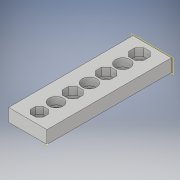
# Autodesk Inventor part: multiplebolts
Saved by Autodesk Inventor 2019 (Build 230136000, 136)
## iProperties
Created: 2018-12-20
Part Number: multiplebolts
Material: Generic
Document SubType Name: Modeling
Designer: assman
Density: 1 g/cm^3
Appearance: Default
Author: assman
## iProperties of the stored document multiplebolts_3DPrint.ipt
Created: 2018-12-20
Part Number: multiplebolts_3DPrint
Material: Generic
Document SubType Name: Modeling
Designer: assman
Density: 1 g/cm^3
Appearance: Default
Author: assman
Autodesk Inventor part; units mm, degrees
ref_plane "YZ Plane" through (0, 0, 0) normal (1, 0, 0) x (0, 1, 0)
ref_plane "XZ Plane" through (0, 0, 0) normal (0, 1, 0) x (-1, 0, 0)
ref_plane "XY Plane" through (0, 0, 0) normal (0, 0, 1) x (1, 0, 0)
sketch "Sketch1" plane through (0, 0, 0) normal (0, 1, 0) x (-1, 0, 0)
  line L0 (15, 0) -> (0, 0)
  line L1 (0, 0) -> (0, -50)
  line L2 (0, -50) -> (15, -50)
  line L3 (15, -50) -> (15, 0)
  dimension "d0" = 15
  dimension "d1" = 50
  constraints: 8 end point, 2 parallel, 1 coincident, 1 horizontal, 1 perpendicular
  measures "d0" distance of L2.end L1.end
  measures "d1" distance of L1.end L0.end
extrude "Extrusion1" add sketch "Sketch1" along normal blind 5
sketch "Sketch2" plane through (0, 5, 0) normal (0, 1, 0) x (1, 0, 0)
  line L0 (-15, 50) -> (-15, 0) construction
  line L1 (-15, 0) -> (0, 0) construction
  line L2 (0, 0) -> (0, 50) construction
  line L3 (0, 50) -> (-15, 50) construction
  line L4 (-15, 50) -> (-15, 0) construction
  line L5 (-15, 0) -> (0, 0) construction
  line L6 (-7.5, 0) -> (-7.5, 50) construction
  line L7 (0, 50) -> (-15, 50) construction
  line L8 (-15, 25) -> (0, 25) construction
  line L9 (-4.9593, 5.6025) -> (-4.9593, 3.4978)
  line L10 (-4.9593, 3.4978) -> (-6.4476, 2.0095)
  line L11 (-6.4476, 2.0095) -> (-8.5524, 2.0095)
  line L12 (-8.5524, 2.0095) -> (-10.0407, 3.4978)
  line L13 (-10.0407, 3.4978) -> (-10.0407, 5.6025)
  line L14 (-10.0407, 5.6025) -> (-8.5524, 7.0908)
  line L15 (-8.5524, 7.0908) -> (-6.4476, 7.0908)
  line L16 (-6.4476, 7.0908) -> (-4.9593, 5.6025)
  line L17 (-15, 2.0095) -> (0, 2.0095) construction
  line L18 (0, 0) -> (0, 50) construction
  line L19 (-10.4, 16.3489) -> (-10.4, 18.7514)
  line L20 (-10.4, 18.7514) -> (-8.7012, 20.4502)
  line L21 (-8.7012, 20.4502) -> (-6.2988, 20.4502)
  line L22 (-6.2988, 20.4502) -> (-4.6, 18.7514)
  line L23 (-4.6, 18.7514) -> (-4.6, 16.3489)
  line L24 (-4.6, 16.3489) -> (-6.2988, 14.6502)
  line L25 (-6.2988, 14.6502) -> (-8.7012, 14.6502)
  line L26 (-8.7012, 14.6502) -> (-10.4, 16.3489)
  line L27 (-7.5, 4.5502) -> (-7.5, 17.5502) construction
  circle A0 centre (-7.5, 11.0502) radius 2.75
  line L28 (-7.5, 17.5502) -> (-7.5, 30.5502) construction
  circle A1 centre (-7.5, 24.0502) radius 2.825
  line L29 (-4.55, 31.7721) -> (-4.55, 29.3282)
  line L30 (-4.55, 29.3282) -> (-6.2781, 27.6002)
  line L31 (-6.2781, 27.6002) -> (-8.7219, 27.6002)
  line L32 (-8.7219, 27.6002) -> (-10.45, 29.3282)
  line L33 (-10.45, 29.3282) -> (-10.45, 31.7721)
  line L34 (-10.45, 31.7721) -> (-8.7219, 33.5002)
  line L35 (-8.7219, 33.5002) -> (-6.2781, 33.5002)
  line L36 (-6.2781, 33.5002) -> (-4.55, 31.7721)
  line L37 (-7.5, 30.5502) -> (-7.5, 43.5502) construction
  circle A2 centre (-7.5, 37.0502) radius 2.85
  line L38 (-4.5, 44.7928) -> (-4.5, 42.3075)
  line L39 (-4.5, 42.3075) -> (-6.2574, 40.5502)
  line L40 (-6.2574, 40.5502) -> (-8.7426, 40.5502)
  line L41 (-8.7426, 40.5502) -> (-10.5, 42.3075)
  line L42 (-10.5, 42.3075) -> (-10.5, 44.7928)
  line L43 (-10.5, 44.7928) -> (-8.7426, 46.5502)
  line L44 (-8.7426, 46.5502) -> (-6.2574, 46.5502)
  line L45 (-6.2574, 46.5502) -> (-4.5, 44.7928)
  line L46 (-15, 46.5502) -> (0, 46.5502) construction
  line L47 (-15, 48.5597) -> (0, 48.5597) construction
  dimension "d12" = 2.0095
  dimension "d14" = 2.5407
  dimension "d15" = 2.9
  dimension "d17" = 5.5
  dimension "d18" = 5.65
  dimension "d19" = 2.95
  dimension "d20" = 5.7
  dimension "d21" = 3
  dimension "d22" = 2.0095
  constraints: 80 end point, 6 point on line, 4 collinear, 4 midpoint, 4 parallel, 3 centre point, 3 perpendicular, 1 coincident, 20 other
  measures "d12" distance between parallel lines of L1 L17
  measures "d14" distance from line of L27.start L10
  measures "d15" distance from line of L27.end L24
  measures "d17" diameter of A0
  measures "d18" diameter of A1
  measures "d19" distance from line of L30 L37.start
  measures "d20" diameter of A2
  measures "d21" distance from line of point (-7.5, 43.55) L39
  measures "d22" distance between parallel lines of L46 L47
ref_plane "Work Plane1" through (-15, 5, -48.5597) normal (0, 0, 1) x (1, 0, 0)
split "Split1" plane through (-15, 5, -48.5597) removes the side toward (0, 0, -1)
extrude "Extrusion2" cut sketch "Sketch2" against normal blind 2.85 contours L9 L10 L11 L12 L13 L14 L15 L16
extrude "Extrusion6" cut sketch "Sketch2" against normal blind 2.85 contours A0
extrude "Extrusion3" cut sketch "Sketch2" against normal blind 3 contours L19 L20 L21 L22 L23 L24 L25 L26
extrude "Extrusion7" cut sketch "Sketch2" against normal blind 3 contours A1
extrude "Extrusion4" cut sketch "Sketch2" against normal blind 3.05 contours L29 L30 L31 L32 L33 L34 L35 L36
extrude "Extrusion5" cut sketch "Sketch2" against normal blind 3.1 contours L38 L39 L40 L41 L42 L43 L44 L45
hole "Hole2" at (-7.5, 5, -4.5502) direction (0, -1, 0) diameter 3.121 end through all thread size "M3.5x0.35" class "6H" standard "ISO Metric profile"
hole "Hole3" at (-7.5, 5, -11.0502) direction (0, -1, 0) diameter 3.121 end through all thread size "M3.5x0.35" class "6H" standard "ISO Metric profile"
hole "Hole4" at (-7.5, 5, -17.5502) direction (0, -1, 0) diameter 3.242 end through all thread size "M4x0.7" class "6H" standard "ISO Metric profile"
hole "Hole5" at (-7.5, 5, -24.0502) direction (0, -1, 0) diameter 3.242 end through all thread size "M4x0.7" class "6H" standard "ISO Metric profile"
hole "Hole6" at (-7.5, 5, -30.5502) direction (0, -1, 0) diameter 3.459 end through all thread size "M4x0.5" class "6H" standard "ISO Metric profile"
extrude "Extrusion8" cut sketch "Sketch2" against normal blind 3.1 contours A2
sketch "Sketch4" plane through (-7.5, 1.9, -37.0502) normal (0, 1, 0) x (1, 0, 0)
  circle A0 centre (0, 0) radius 2.85 construction
  line L0 (0, 0) -> (0, 2.85) construction
  line L1 (-1.5605, -0.6464) -> (-1.5605, 0.6464)
  line L2 (-1.5605, 0.6464) -> (-0.6464, 1.5605)
  line L3 (-0.6464, 1.5605) -> (0.6464, 1.5605)
  line L4 (0.6464, 1.5605) -> (1.5605, 0.6464)
  line L5 (1.5605, 0.6464) -> (1.5605, -0.6464)
  line L6 (1.5605, -0.6464) -> (0.6464, -1.5605)
  line L7 (0.6464, -1.5605) -> (-0.6464, -1.5605)
  line L8 (-0.6464, -1.5605) -> (-1.5605, -0.6464)
  point P0 (7.5, -37.0502)
  dimension "d81" = 1.5605
  constraints: 18 end point, 1 coincident, 1 parallel, 1 vertical, 1 vertical alignment, 18 other
  measures "d81" distance from line of L0.start L8
sketch "Sketch5" plane through (0, 0, 0) normal (0, -1, 0) x (1, 0, 0)
  point P0 (0, 0)
extrude "Extrusion9" cut sketch "Sketch4" against normal blind 3.1
sketch "Sketch6" plane through (0, 1.9, 0) normal (0, 1, 0) x (1, 0, 0)
  line L0 (-4.5, 44.7928) -> (-4.5, 42.3075) construction
  line L1 (-6.2574, 46.5502) -> (-4.5, 44.7928) construction
  line L2 (-8.7426, 46.5502) -> (-6.2574, 46.5502) construction
  line L3 (-10.5, 44.7928) -> (-8.7426, 46.5502) construction
  line L4 (-10.5, 42.3075) -> (-10.5, 44.7928) construction
  line L5 (-8.7426, 40.5502) -> (-10.5, 42.3075) construction
  line L6 (-6.2574, 40.5502) -> (-8.7426, 40.5502) construction
  line L7 (-4.5, 42.3075) -> (-6.2574, 40.5502) construction
  line L8 (-4.5, 42.3075) -> (-6.2574, 40.5502) construction
  line L9 (-4.5, 42.3075) -> (-10.5, 44.7928) construction
  line L10 (-10.5, 42.3075) -> (-10.5, 44.7928) construction
  line L11 (-6.2574, 46.5502) -> (-4.5, 44.7928) construction
  line L12 (-10.5, 42.3075) -> (-4.5, 44.7928) construction
  line L13 (-7.5, 43.5502) -> (-7.5, 46.5502) construction
  line L14 (-7.5, 46.5502) -> (-7.5, 40.5502) construction
  line L15 (-6.2574, 40.5502) -> (-8.7426, 40.5502) construction
  line L16 (-9.2105, 42.8416) -> (-9.2105, 44.2587)
  line L17 (-9.2105, 44.2587) -> (-8.2085, 45.2607)
  line L18 (-8.2085, 45.2607) -> (-6.7915, 45.2607)
  line L19 (-6.7915, 45.2607) -> (-5.7895, 44.2587)
  line L20 (-5.7895, 44.2587) -> (-5.7895, 42.8416)
  line L21 (-5.7895, 42.8416) -> (-6.7915, 41.8397)
  line L22 (-6.7915, 41.8397) -> (-8.2085, 41.8397)
  line L23 (-8.2085, 41.8397) -> (-9.2105, 42.8416)
  point P0 (0, 0)
  dimension "d84" = 1.7105
  constraints: 24 end point, 3 midpoint, 2 point on line, 1 coincident, 17 other
  measures "d84" distance from line of L13.start L23
extrude "Extrusion10" cut sketch "Sketch6" against normal blind 3.1
thread "Thread2" size "M3.5x0.6" class "6H" standard "ANSI Metric M Profile" full length
thread "Thread3" size "M3.5x0.6" class "6H" standard "ANSI Metric M Profile" full length
sketch "Sketch8" plane through (-7.5, 2.15, -11.0502) normal (1, 0, 0) x (0, 0, 1)
  line L0 (1.5605, 0) -> (1.5605, 2.15)
  line L1 (1.5605, 2.15) -> (1.1156, 2.15)
  line L2 (1.1156, 2.15) -> (1.1156, 0)
  line L3 (1.1156, 0) -> (1.5605, 0)
  line L4 (0, -3.85) -> (0, 3.15) projected
  constraints: 8 end point
revolve "Revolution1" add sketch "Sketch8" angle 360 about axis through (-7.5, 2.15, -11.0502) along (0, -1, 0) separate body
sketch "Sketch7" plane through (-7.5, 2.15, -9.4897) normal (-1, 0, 0) x (0, -1, 0)
  line L0 (-0.3501, -0.0305) -> (-0.3001, -0.0305) construction
  line L1 (0.0499, -0.4147) -> (-0.0001, -0.5108) construction
  line L2 (-0.6001, -0.5108) -> (-0.6501, -0.4147) construction
  line L3 (-0.2501, -0.0305) -> (-0.3001, 0.0655) construction
  line L4 (-0.3001, 0.0655) -> (-0.3501, -0.0305) construction
  line L5 (-0.6001, -0.5108) -> (-0.5501, -0.4147) construction
  line L6 (-0.2501, -0.0305) -> (-0.0501, -0.4147)
  line L7 (-0.6501, -0.4147) -> (-0.5501, -0.4147) construction
  arc A0 (-0.6501, -0.4147) -> (-0.6001, -0.445) centre (-0.6001, -0.3887) ccw construction
  line L8 (0.0499, -0.4147) -> (-0.0501, -0.4147) construction
  line L9 (-0.6001, -0.5108) -> (-0.6001, -0.4147) construction
  line L10 (-0.0001, -0.5108) -> (-0.0001, -0.4147) construction
  line L11 (-0.3001, 0.0655) -> (-0.3001, -0.0002) construction
  line L12 (-0.6001, -0.445) -> (-0.0001, -0.445)
  arc A1 (-0.6001, -0.445) -> (-0.5501, -0.4147) centre (-0.6001, -0.3887) ccw
  line L13 (-0.0501, -0.4147) -> (-0.0001, -0.5108) construction
  line L14 (-0.5501, -0.4147) -> (-0.3501, -0.0305)
  line L15 (-0.0001, -0.0002) -> (-0.0001, 0.0177)
  line L16 (-0.0001, 0.0177) -> (-0.0001, -0.0002)
  line L17 (-0.0001, -0.0002) -> (0.0334, -0.0002)
  arc A2 (-0.0501, -0.4147) -> (-0.0001, -0.445) centre (-0.0001, -0.3887) ccw
  arc A3 (-0.0001, -0.445) -> (0.0499, -0.4147) centre (-0.0001, -0.3887) ccw construction
  arc A4 (-0.3001, -0.0002) -> (-0.3501, -0.0305) centre (-0.3001, -0.0565) ccw
  arc A5 (-0.2501, -0.0305) -> (-0.3001, -0.0002) centre (-0.3001, -0.0565) ccw
  line L18 (-0.3001, -0.0002) -> (-0.3001, -0.0305) construction
  line L19 (-0.3001, -0.0305) -> (-0.2501, -0.0305) construction
  dimension "d93" = 55
  dimension "d94" = 0.096
  dimension "d95" = 0.096
  dimension "Sketch7_ThreadOffset" = 0
  dimension "Sketch7_MajorRadius" = 0.4449
  dimension "d98" = 0.6
  dimension "Sketch7_MinorRadius" = 0
  constraints: 40 end point, 12 point on circle, 10 parallel, 8 tangent, 6 centre point, 6 collinear, 2 midpoint, 2 point on line, 1 horizontal, 1 perpendicular, 3 other
  measures "d93" angle of L6 L14
  measures "d94" distance of L3.end L0.end
  measures "d95" distance of L1.end L10.end
  measures "Sketch7_ThreadOffset" distance between parallel lines of L15 L10
  measures "Sketch7_MajorRadius" distance from line of L12 L15.start
  measures "d98" distance from line of L1.end L9
  measures "Sketch7_MinorRadius" distance edge to line of A5 L17
coil "Coil1" sketch "Sketch7" operation cut axis through (-7.5, 2.15, -11.0502) along (0, -1, 0) pitch 0.6006 turns 5.577756 hand right bodies 2
sketch "Sketch10" plane through (-7.5, 2, -24.0502) normal (1, 0, 0) x (0, 0, 1)
  line L0 (1.621, 0) -> (1.621, 2)
  line L1 (1.621, 2) -> (1.1761, 2)
  line L2 (1.1761, 2) -> (1.1761, 0)
  line L3 (1.1761, 0) -> (1.621, 0)
  line L4 (0, -4.04) -> (0, 3.24) projected
  constraints: 8 end point
revolve "Revolution2" add sketch "Sketch10" angle 360 about axis through (-7.5, 2, -24.0502) along (0, -1, 0) separate body
sketch "Sketch9" plane through (-7.5, 2, -22.4292) normal (-1, 0, 0) x (0, -1, 0)
  line L0 (-0.3501, -0.0305) -> (-0.3001, -0.0305) construction
  line L1 (0.0499, -0.4147) -> (-0.0001, -0.5108) construction
  line L2 (-0.6001, -0.5108) -> (-0.6501, -0.4147) construction
  line L3 (-0.2501, -0.0305) -> (-0.3001, 0.0655) construction
  line L4 (-0.3001, 0.0655) -> (-0.3501, -0.0305) construction
  line L5 (-0.6001, -0.5108) -> (-0.5501, -0.4147) construction
  line L6 (-0.2501, -0.0305) -> (-0.0501, -0.4147)
  line L7 (-0.6501, -0.4147) -> (-0.5501, -0.4147) construction
  arc A0 (-0.6501, -0.4147) -> (-0.6001, -0.445) centre (-0.6001, -0.3887) ccw construction
  line L8 (0.0499, -0.4147) -> (-0.0501, -0.4147) construction
  line L9 (-0.6001, -0.5108) -> (-0.6001, -0.4147) construction
  line L10 (-0.0001, -0.5108) -> (-0.0001, -0.4147) construction
  line L11 (-0.3001, 0.0655) -> (-0.3001, -0.0002) construction
  line L12 (-0.6001, -0.445) -> (-0.0001, -0.445)
  arc A1 (-0.6001, -0.445) -> (-0.5501, -0.4147) centre (-0.6001, -0.3887) ccw
  line L13 (-0.0501, -0.4147) -> (-0.0001, -0.5108) construction
  line L14 (-0.5501, -0.4147) -> (-0.3501, -0.0305)
  line L15 (-0.0001, -0.0002) -> (-0.0001, 0.0177)
  line L16 (-0.0001, 0.0177) -> (-0.0001, -0.0002)
  line L17 (-0.0001, -0.0002) -> (0.0334, -0.0002)
  arc A2 (-0.0501, -0.4147) -> (-0.0001, -0.445) centre (-0.0001, -0.3887) ccw
  arc A3 (-0.0001, -0.445) -> (0.0499, -0.4147) centre (-0.0001, -0.3887) ccw construction
  arc A4 (-0.3001, -0.0002) -> (-0.3501, -0.0305) centre (-0.3001, -0.0565) ccw
  arc A5 (-0.2501, -0.0305) -> (-0.3001, -0.0002) centre (-0.3001, -0.0565) ccw
  line L18 (-0.3001, -0.0002) -> (-0.3001, -0.0305) construction
  line L19 (-0.3001, -0.0305) -> (-0.2501, -0.0305) construction
  dimension "d111" = 55
  dimension "d112" = 0.096
  dimension "d113" = 0.096
  dimension "Sketch9_ThreadOffset" = 0
  dimension "Sketch9_MajorRadius" = 0.4449
  dimension "d116" = 0.6
  dimension "Sketch9_MinorRadius" = 0
  constraints: 40 end point, 12 point on circle, 10 parallel, 8 tangent, 6 centre point, 6 collinear, 2 midpoint, 2 point on line, 1 horizontal, 1 perpendicular, 3 other
  measures "d111" angle of L6 L14
  measures "d112" distance of L3.end L0.end
  measures "d113" distance of L1.end L10.end
  measures "Sketch9_ThreadOffset" distance between parallel lines of L15 L10
  measures "Sketch9_MajorRadius" distance from line of L12 L15.start
  measures "d116" distance from line of L1.end L9
  measures "Sketch9_MinorRadius" distance edge to line of A5 L17
coil "Coil2" sketch "Sketch9" operation cut axis through (-7.5, 2, -24.0502) along (0, -1, 0) pitch 0.6006 turns 5.328005 hand right bodies 3
equation "\"d22\" = d12"
equation "\"d93\" = d100"
equation "\"d94\" = 0.160083 * Sketch7_Pitch"
equation "\"d95\" = 0.160083 * Sketch7_Pitch"
equation "\"d98\" = Sketch7_Pitch"
equation "\"d111\" = d118"
equation "\"d112\" = 0.160083 * Sketch9_Pitch"
equation "\"d113\" = 0.160083 * Sketch9_Pitch"
equation "\"d116\" = Sketch9_Pitch"
equation "\"d100\" = 55deg"
equation "\"Sketch7_Pitch\" = 0.6"
equation "\"d118\" = 55deg"
equation "\"Sketch9_Pitch\" = 0.6"
body "Solid1"
body "Solid2"
body "Solid3"
